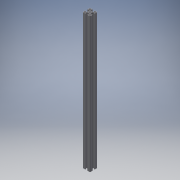
# Autodesk Inventor part: Propile_37
Saved by Autodesk Inventor 2019 (Build 230136000, 136)
## iProperties
Created: 2019-04-05
Part Number: Propile_37
Material: 일반
Document SubType Name: Modeling
Designer: hinmo
Density: 1 g/cm^3
Appearance: 기본값
Author: hinmo
Autodesk Inventor part; units mm, degrees
ref_plane "YZ Plane" through (0, 0, 0) normal (1, 0, 0) x (0, 1, 0)
ref_plane "XZ Plane" through (0, 0, 0) normal (0, 1, 0) x (-1, 0, 0)
ref_plane "XY Plane" through (0, 0, 0) normal (0, 0, 1) x (1, 0, 0)
sketch "스케치1" plane through (0, 0, 0) normal (0, 1, 0) x (-1, 0, 0)
  circle A0 centre (7, -7) radius 2
  circle A1 centre (-7, -7) radius 2
  circle A2 centre (0, 0) radius 2.15
  line L0 (2.65, 10) -> (2.65, 8.5)
  line L1 (2.65, 8.5) -> (4.15, 8.5)
  line L2 (4.15, 8.5) -> (4.15, 4.9)
  arc A3 (-4.15, 4.9) -> (4.15, 4.9) centre (0, 9.482) ccw
  line L3 (-4.15, 4.9) -> (-4.15, 8.5)
  line L4 (-4.15, 8.5) -> (-2.65, 8.5)
  line L5 (-2.65, 8.5) -> (-2.65, 10)
  line L6 (-2.65, 10) -> (-9, 10)
  arc A4 (-9, 10) -> (-10, 9) centre (-9, 9) ccw
  line L7 (-10, 9) -> (-10, 2.65)
  line L8 (-10, 2.65) -> (-8.5, 2.65)
  line L9 (-8.5, 2.65) -> (-8.5, 4.15)
  line L10 (-8.5, 4.15) -> (-4.9, 4.15)
  arc A5 (-4.9, -4.15) -> (-4.9, 4.15) centre (-9.482, 0) ccw
  line L11 (-4.9, -4.15) -> (-8.5, -4.15)
  line L12 (-8.5, -4.15) -> (-8.5, -2.65)
  line L13 (-8.5, -2.65) -> (-10, -2.65)
  line L14 (-10, -2.65) -> (-10, -9)
  arc A6 (-10, -9) -> (-9, -10) centre (-9, -9) ccw
  line L15 (-9, -10) -> (-2.65, -10)
  line L16 (-2.65, -10) -> (-2.65, -8.5)
  line L17 (-2.65, -8.5) -> (-4.15, -8.5)
  line L18 (-4.15, -8.5) -> (-4.15, -4.9)
  arc A7 (4.15, -4.9) -> (-4.15, -4.9) centre (0, -9.482) ccw
  line L19 (4.15, -4.9) -> (4.15, -8.5)
  line L20 (4.15, -8.5) -> (2.65, -8.5)
  line L21 (2.65, -8.5) -> (2.65, -10)
  line L22 (2.65, -10) -> (9, -10)
  arc A8 (9, -10) -> (10, -9) centre (9, -9) ccw
  line L23 (10, -9) -> (10, -2.65)
  line L24 (10, -2.65) -> (8.5, -2.65)
  line L25 (8.5, -2.65) -> (8.5, -4.15)
  line L26 (8.5, -4.15) -> (4.9, -4.15)
  arc A9 (4.9, 4.15) -> (4.9, -4.15) centre (9.482, 0) ccw
  line L27 (4.9, 4.15) -> (8.5, 4.15)
  line L28 (8.5, 4.15) -> (8.5, 2.65)
  line L29 (8.5, 2.65) -> (10, 2.65)
  line L30 (10, 2.65) -> (10, 9)
  arc A10 (10, 9) -> (9, 10) centre (9, 9) ccw
  line L31 (9, 10) -> (2.65, 10)
  circle A11 centre (7, 7) radius 2
  circle A12 centre (-7, 7) radius 2
  constraints: 64 end point, 16 point on circle, 13 centre point
extrude "돌출1" add sketch "스케치1" along normal blind 370
